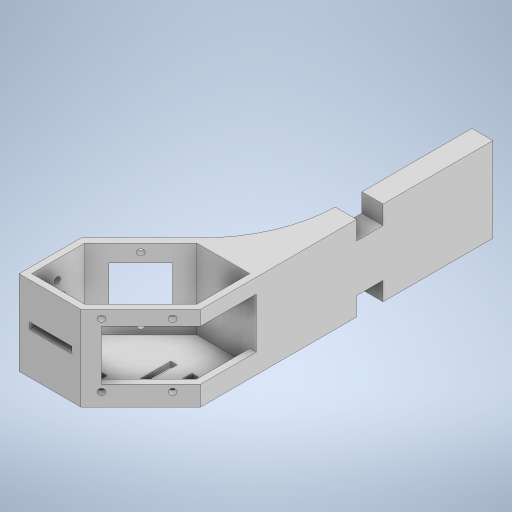
# Autodesk Inventor part: tactic2 chassis1
Saved by Autodesk Inventor 2024 (Build 280153000, 153)
## iProperties
Created: 2024-11-08
Part Number: tactic2 chassis1
Material: Generic
Document SubType Name: Modeling
Designer: Williamow
Density: 1 g/cm^3
Appearance: Default
Author: Williamow
Autodesk Inventor part; units mm, degrees
ref_plane "YZ Plane" through (0, 0, 0) normal (1, 0, 0) x (0, 1, 0)
ref_plane "XZ Plane" through (0, 0, 0) normal (0, 1, 0) x (-1, 0, 0)
ref_plane "XY Plane" through (0, 0, 0) normal (0, 0, 1) x (1, 0, 0)
sketch "Sketch1" plane through (0, 0, 0) normal (0, 1, 0) x (-1, 0, 0)
  line L0 (10.6066, 0) -> (0, -10.6066)
  line L1 (0, -10.6066) -> (0, -20.6066)
  line L2 (0, -20.6066) -> (10, -20.6066)
  line L3 (10, -20.6066) -> (20.6066, -10)
  line L4 (20.6066, -10) -> (20.6066, 0)
  line L5 (20.6066, 0) -> (10.6066, 0)
  line L6 (21.8066, 1.2) -> (21.8066, -10.4971)
  line L7 (21.8066, -10.4971) -> (10.4971, -21.8066)
  line L8 (10.4971, -21.8066) -> (-1.2, -21.8066)
  line L9 (-1.2, -21.8066) -> (-1.2, -10.1095)
  line L10 (-1.2, -10.1095) -> (10.1095, 1.2)
  line L11 (10.1095, 1.2) -> (21.8066, 1.2)
  line L12 (-1.2, -21.8066) -> (-1.2, -40.3889)
  line L13 (-1.2, -40.3889) -> (2.8, -40.3889)
  arc A0 (10.4971, -21.8066) -> (2.8, -40.3889) centre (29.0794, -40.3889) ccw
  line L14 (4.8083, -4.1012) -> (5.5154, -4.8083) construction
  line L15 (5.5154, -4.8083) -> (13.9559, -4.8083) construction
  line L16 (5.5154, -4.8083) -> (5.5154, -15.0259) construction
  line L17 (-1.2, -40.3889) -> (2.8, -40.3889)
  line L18 (2.8, -40.3889) -> (2.8, -65.3889)
  line L19 (2.8, -65.3889) -> (-1.2, -65.3889)
  line L20 (-1.2, -65.3889) -> (-1.2, -40.3889)
  point P0 (0, 0)
  point P1 (4.4548, -4.4548)
  dimension "d0" = 135
  dimension "d2" = 15
  dimension "d3" = 10
  dimension "d4" = 10
  dimension "d5" = 10
  dimension "d6" = 1.2
  dimension "d29" = 4
  dimension "d44" = 1
  dimension "d45" = 0.5
  dimension "d52" = 25
  constraints: 42 end point, 7 perpendicular, 4 parallel, 3 horizontal, 3 vertical, 2 point on circle, 2 vertical alignment, 1 centre point, 1 horizontal alignment, 1 line through centre, 1 midpoint, 1 point on line, 1 tangent, 5 other
  measures "d0" angle of L5 L0
  measures "d2" distance of L0.start L0.end
  measures "d3" distance of L0.end L1.end
  measures "d4" distance of L0.start L4.end
  measures "d5" distance of L1.end L2.end
  measures "d6" distance between parallel lines of L4 L6
  measures "d29" distance of L12.end L13.end
  measures "d44" distance of L14.start L14.end
  measures "d45" distance of point (4.455, -4.455) L14.start
  measures "d52" distance of L17.end L18.end
extrude "Extrusion1" add sketch "Sketch1" along normal blind 1 contours L5 L4 L3 L2 L1 L0
extrude "Extrusion2" add sketch "Sketch1" along normal blind 16
sketch "Sketch2" plane through (1.2, 0, -10.1095) normal (0.7071, 0, 0.7071) x (0.7071, 0, -0.7071)
  line L0 (-15.9941, 0) -> (0, 0) projected
  line L1 (0, 0) -> (0, 16) projected
  line L2 (-15.9941, 16) -> (0, 16) projected
  line L3 (-15.9941, 0) -> (-15.9941, 16) projected
  line L4 (-13.2471, 13.25) -> (-3.7471, 13.25)
  line L5 (-3.7471, 13.25) -> (-3.7471, 3.75)
  line L6 (-3.7471, 3.75) -> (-13.2471, 3.75)
  line L7 (-13.2471, 3.75) -> (-13.2471, 13.25)
  circle A0 centre (-13.2471, 14.5) radius 0.6
  circle A1 centre (-3.7471, 14.5) radius 0.6
  circle A2 centre (-3.7471, 2.5) radius 0.6
  circle A3 centre (-13.2471, 2.5) radius 0.6
  point P0 (-7.9971, 0)
  point P1 (-8.4971, 13.25)
  point P2 (-7.9971, 16)
  point P3 (-13.2471, 8.5)
  point P4 (-15.9941, 8)
  point P5 (-8.4971, 0)
  point P6 (-8.4971, 0)
  point P7 (-8.4971, 0)
  dimension "d11" = 0.5
  dimension "d12" = 9.5
  dimension "d13" = 6
  dimension "d14" = 6
  dimension "d15" = 1.2
  constraints: 8 end point, 5 vertical alignment, 4 centre point, 4 midpoint, 3 equal radius, 2 horizontal alignment, 2 parallel, 2 perpendicular, 1 horizontal
  measures "d11" vertical distance of point (-13.247, 8.5) point (-15.994, 8)
  measures "d12" distance of L4.start L4.end
  measures "d13" distance of A0.centre point (-13.247, 8.5)
  measures "d14" distance of A3.centre point (-13.247, 8.5)
  measures "d15" diameter of A1
extrude "Extrusion3" cut sketch "Sketch2" against normal blind 2 contours L4 L5 L6 L7 | A0 | A1 | A2 | A3
sketch "Sketch3" plane through (1.2, 0, -10.1095) normal (1, 0, 0) x (0, 0, -1)
  line L0 (-9.3671, 13.25) -> (-2.6496, 13.25) projected
  line L1 (-2.6496, 3.75) -> (-9.3671, 3.75) projected
  line L2 (-2.6496, 3.75) -> (10.4971, 3.75)
  line L3 (10.4971, 3.75) -> (10.4971, 13.25)
  line L4 (10.4971, 13.25) -> (-2.6496, 13.25)
  line L5 (-2.6496, 13.25) -> (-2.6496, 3.75)
  line L6 (10.4971, 1) -> (10.4971, 16) projected
  line L7 (0, 16) -> (55.2794, 16) projected
  line L8 (55.2794, 0) -> (55.2794, 16) projected
  line L9 (0, 0) -> (55.2794, 0) projected
  line L10 (34.4971, 0) -> (29.4971, 0)
  line L11 (29.4971, 0) -> (29.4971, 3.5)
  line L12 (29.4971, 3.5) -> (34.4971, 3.5)
  line L13 (34.4971, 3.5) -> (34.4971, 0)
  line L14 (29.4971, 16) -> (34.4971, 16)
  line L15 (34.4971, 16) -> (34.4971, 12.5)
  line L16 (34.4971, 12.5) -> (29.4971, 12.5)
  line L17 (29.4971, 12.5) -> (29.4971, 16)
  point P0 (-10.1095, 0)
  point P1 (55.2794, 8)
  dimension "d59" = 5
  dimension "d60" = 9
  dimension "d66" = 20.7823
  constraints: 24 end point, 6 parallel, 4 point on line, 3 horizontal, 3 perpendicular, 1 coincident, 1 collinear, 1 midpoint, 1 vertical alignment
  measures "d59" distance of L10.start L10.end
  measures "d60" distance between parallel lines of L16 L12
  measures "d66" horizontal distance of point (55.279, 8) L14.end
extrude "Extrusion4" cut sketch "Sketch3" against normal up to next
sketch "Sketch4" plane through (-21.8066, 0, -10.4971) normal (-0.7071, 0, -0.7071) x (-0.7071, 0, 0.7071)
  line L0 (-15.9941, 0) -> (0, 0) projected
  line L1 (0, 0) -> (0, 16) projected
  line L2 (-15.9941, 16) -> (0, 16) projected
  line L3 (-15.9941, 0) -> (-15.9941, 16) projected
  line L4 (-12.2471, 12.75) -> (-3.7471, 12.75)
  line L5 (-3.7471, 12.75) -> (-3.7471, 4.25)
  line L6 (-3.7471, 4.25) -> (-12.2471, 4.25)
  line L7 (-12.2471, 4.25) -> (-12.2471, 12.75)
  circle A0 centre (-7.9971, 14.5) radius 0.6
  circle A1 centre (-7.9971, 2.5) radius 0.6
  point P0 (-7.9971, 0)
  point P1 (-7.9971, 12.75)
  point P2 (-7.9971, 16)
  point P3 (0, 8)
  point P4 (-3.7471, 8.5)
  point P5 (-12.2471, 8.5)
  dimension "d21" = 0.5
  dimension "d22" = 8.5
  dimension "d23" = 6
  dimension "d24" = 6
  dimension "d25" = 1.2
  constraints: 8 end point, 5 midpoint, 3 vertical alignment, 2 centre point, 2 parallel, 2 perpendicular, 1 equal radius, 1 horizontal
  measures "d21" vertical distance of point (0, 8) point (-3.747, 8.5)
  measures "d22" distance of L4.start L4.end
  measures "d23" vertical distance of point (-12.247, 8.5) A0.centre
  measures "d24" vertical distance of A1.centre point (-12.247, 8.5)
  measures "d25" diameter of A1
extrude "Extrusion5" cut sketch "Sketch4" against normal blind 2 contours L4 L5 L6 L7 | A0 | A1
sketch "Sketch5" plane through (-21.8066, 0, -10.4971) normal (-1, 0, 0) x (0, 0, 1)
  line L0 (10.4971, 1) -> (10.4971, 16) projected
  circle A0 centre (5.6887, 8.5) radius 2
  circle A1 centre (5.6887, 12.5) radius 0.6
  circle A2 centre (5.6887, 4.5) radius 0.6
  circle A3 centre (9.6887, 8.5) radius 0.6
  point P0 (10.4971, 0)
  point P1 (10.4971, 8.5)
  point P2 (5.6887, 0)
  point P3 (5.6887, 0)
  point P4 (5.6887, 0)
  dimension "d30" = 4
  dimension "d31" = 1.2
  dimension "d32" = 4
  dimension "d33" = 4
  dimension "d34" = 4
  constraints: 4 centre point, 3 vertical alignment, 2 equal radius, 2 horizontal alignment, 1 midpoint
  measures "d30" diameter of A0
  measures "d31" diameter of A1
  measures "d32" distance of A1.centre A0.centre
  measures "d33" distance of A2.centre A0.centre
  measures "d34" distance of A3.centre A0.centre
extrude "Extrusion6" cut sketch "Sketch5" against normal blind 2
sketch "Sketch6" plane through (0, 0, 0) normal (0, -1, 0) x (1, 0, 0)
  line L0 (-21.8066, -6.8083) -> (-21.8066, -2.8083) projected
  line L1 (-11.8066, -7.4083) -> (-19.8066, -7.4083)
  line L2 (-19.8066, -7.4083) -> (-19.8066, -6.2083)
  line L3 (-19.8066, -6.2083) -> (-11.8066, -6.2083)
  line L4 (-11.8066, -6.2083) -> (-11.8066, -7.4083)
  line L5 (-11.8066, -3.4083) -> (-19.8066, -3.4083)
  line L6 (-19.8066, -3.4083) -> (-19.8066, -2.2083)
  line L7 (-19.8066, -2.2083) -> (-11.8066, -2.2083)
  line L8 (-11.8066, -2.2083) -> (-11.8066, -3.4083)
  line L9 (-15.8066, -6.2083) -> (-15.8066, -3.4083) construction
  line L10 (-5.5154, -4.8083) -> (-13.9559, -4.8083) construction
  line L11 (-5.5154, -4.8083) -> (-5.5154, -15.0259) construction
  line L12 (-8.1154, -13.8083) -> (-6.9154, -13.8083)
  line L13 (-6.9154, -13.8083) -> (-6.9154, -7.8083)
  line L14 (-6.9154, -7.8083) -> (-8.1154, -7.8083)
  line L15 (-8.1154, -7.8083) -> (-8.1154, -13.8083)
  line L16 (-4.1154, -13.8083) -> (-2.9154, -13.8083)
  line L17 (-2.9154, -13.8083) -> (-2.9154, -7.8083)
  line L18 (-2.9154, -7.8083) -> (-4.1154, -7.8083)
  line L19 (-4.1154, -7.8083) -> (-4.1154, -13.8083)
  line L20 (-4.1154, -10.8083) -> (-6.9154, -10.8083) construction
  line L21 (-11.8066, -5.4083) -> (-19.8066, -5.4083)
  line L22 (-19.8066, -5.4083) -> (-19.8066, -4.2083)
  line L23 (-19.8066, -4.2083) -> (-11.8066, -4.2083)
  line L24 (-11.8066, -4.2083) -> (-11.8066, -5.4083)
  line L25 (-5.6154, -7.8083) -> (-5.4154, -7.8083)
  line L26 (-5.4154, -7.8083) -> (-5.4154, -13.8083)
  line L27 (-5.4154, -13.8083) -> (-5.6154, -13.8083)
  line L28 (-5.6154, -13.8083) -> (-5.6154, -7.8083)
  point P0 (0, 0)
  point P1 (-21.8066, -4.8083)
  point P2 (-19.8066, -2.8083)
  point P3 (-19.8066, -6.8083)
  point P4 (-15.8066, -7.4083)
  point P5 (-15.8066, -4.8083)
  point P6 (-5.5154, -10.8083)
  point P7 (-3.5154, -13.8083)
  point P8 (-7.5154, -13.8083)
  point P9 (-19.8066, -4.8083)
  point P10 (-5.5154, -7.8083)
  dimension "d38" = 1.2
  dimension "d39" = 4
  dimension "d40" = 8
  dimension "d41" = 6
  dimension "d46" = 1.2
  dimension "d47" = 6
  dimension "d48" = 4
  dimension "d49" = 3
  dimension "d51" = 1.3
  dimension "d62" = 1.2
  constraints: 52 end point, 14 midpoint, 12 parallel, 6 horizontal, 6 perpendicular, 4 horizontal alignment, 4 point on line, 4 vertical alignment, 2 collinear
  measures "d38" distance of L3.end L1.start
  measures "d39" distance of point (-19.807, -2.808) point (-19.807, -6.808)
  measures "d40" distance of L1.start L1.end
  measures "d41" horizontal distance of L0.start point (-15.807, -7.408)
  measures "d46" distance of L12.start L12.end
  measures "d47" distance of L14.end L12.start
  measures "d48" distance of point (-3.515, -13.808) point (-7.515, -13.808)
  measures "d49" distance from line of L14.end L10
  measures "d51" distance of L13.end L25.start
  measures "d62" distance of L21.end L22.end
extrude "Extrusion7" cut sketch "Sketch6" against normal blind 25.4 contours L15 L14 L13 L12 | L19 L18 L17 L16 | L21 L22 L23 L24
sketch "Sketch7" plane through (-21.8066, 0, 1.2) normal (0, 0, 1) x (1, 0, 0)
  line L0 (2, 0) -> (10, 0) projected
  line L1 (0, 6.5) -> (0, 10.5) projected
  line L2 (2, 9.1) -> (10, 9.1)
  line L3 (10, 9.1) -> (10, 7.9)
  line L4 (10, 7.9) -> (2, 7.9)
  line L5 (2, 7.9) -> (2, 9.1)
  point P0 (21.8066, 0)
  point P1 (2, 8.5)
  point P2 (0, 8.5)
  dimension "d63" = 1.2
  constraints: 8 end point, 2 midpoint, 2 parallel, 2 vertical alignment, 1 horizontal, 1 horizontal alignment, 1 perpendicular
  measures "d63" distance of L4.end L2.start
extrude "Extrusion8" cut sketch "Sketch7" against normal up to next
body "Solid1"
